Under Camera 2 (Autodesk Fusion 360 design; units mm, degrees)
Autodesk Fusion 360 part; units mm, degrees
note: some values were not read from the file. Chosen so that the rebuilt part matches the saved one: a direction. Set by a fixed rule: which sketch regions a step uses.
sketch "Sketch1" plane through (0, -227.1998, 566.5) normal (1, 0, 0) x (0, 1, 0) in component "Under Cam"
  line L0 (-26, -3.5) -> (12.5005, -3.5)
  line L1 (12.5005, -3.5) -> (4.8799, -38.213)
  line L2 (4.8799, -38.213) -> (-8.0595, -38.213)
  line L3 (-8.0595, -38.213) -> (-8.0595, -43.5)
  line L4 (-8.0595, -43.5) -> (-17.1111, -43.5)
  line L5 (-17.1111, -43.5) -> (-26, -3.5)
  dimension "d394" = 40
  dimension "d403" = 0
  dimension "d404" = 0
  dimension "d405" = 0
  dimension "d406" = 0
  dimension "d415" = 0
  dimension "d416" = 0
  dimension "d417" = 0
  dimension "d418" = 0
  dimension "d423" = 0
  dimension "d424" = 0
  dimension "d425" = 0
  dimension "d426" = 0
  dimension "d432" = 0
  dimension "d433" = 0
  dimension "d434" = 0
  dimension "d435" = 0
  dimension "d440" = 0
  dimension "d441" = 0
  dimension "d442" = 0
  dimension "d443" = 0
  constraint horizontal L0
  constraint parallel L0 L2
  constraint perpendicular L2 L3
  constraint perpendicular L3 L4
  measures "d394" distance of L0 L4
extrude "Extrude1" add sketch "Sketch1" against normal blind 32 makes body 1 in component "Under Cam"
ref_plane "WorkPlane2" through (-16, -253.2593, 525.6435) normal (0, 1, 0) x (0, 0, -1) in component "Under Cam"
sketch "Sketch2" plane through (-71.456, -253.2593, 540.4111) normal (0, 1, 0) x (1, 0, 0) in component "Under Cam"
  line L0 (71.456, 17.4112) -> (71.456, -22.5888)
  line L1 (71.456, -22.5888) -> (39.456, -22.5888)
  line L2 (39.456, -22.5888) -> (39.456, 17.4112)
  line L3 (39.456, 17.4112) -> (71.456, 17.4112)
  line L4 (41.456, -21.5888) -> (69.456, -21.5888)
  line L5 (69.456, -21.5888) -> (69.456, 17.4112)
  line L6 (69.456, 17.4112) -> (41.456, 17.4112)
  line L7 (41.456, 17.4112) -> (41.456, -21.5888)
  line L8 (41.456, -21.5888) -> (69.456, -21.5888)
  line L9 (69.456, -21.5888) -> (69.456, -22.5888)
  line L10 (69.456, -22.5888) -> (41.456, -22.5888)
  line L11 (41.456, -22.5888) -> (41.456, -21.5888)
  line L12 (41.456, -21.5888) -> (41.456, -22.5888)
  line L13 (69.456, -21.5888) -> (69.456, -22.5888)
  dimension "d273" = 2
  dimension "d274" = 2
  dimension "d275" = 1
  constraint horizontal L4
  constraint vertical L5
  constraint horizontal L6
  constraint vertical L7
  constraint coincident L3 L5.end
  constraint horizontal L8
  constraint vertical L9
  constraint horizontal L10
  constraint vertical L11
  constraint coincident L1 L9.end
  constraint perpendicular L10 L13
  measures "d273" horizontal distance of L1.end L4.start
  measures "d274" horizontal distance of L0.end L4.end
  measures "d275" vertical distance of L0.end L4.end
extrude "Extrude2" cut sketch "Sketch2" along normal blind 10 contours L3 L4 L5 L6 L7 L8 | L1 L4 L8 L9 L10 L11 L12 L13 bodies 1 in component "Under Cam"
sketch "Sketch8" plane through (0, 0, 563) normal (0, 0, 1) x (-1, 0, 0) in component "Under Cam"
  line L0 (0, 253.1998) -> (0, 214.6993)
  line L1 (0, 214.6993) -> (32, 214.6993)
  line L2 (32, 214.6993) -> (32, 253.1998)
  line L3 (2, 253.1998) -> (0, 253.1998)
  line L4 (20, 214.6965) -> (20, 253.2026) construction
  circle A0 centre (20, 226.9495) radius 0.75
  circle A1 centre (20, 240.9495) radius 0.75
  line L5 (20, 233.9495) -> (0, 233.9495) construction
  line L6 (30, 253.1998) -> (30, 243.2593)
  line L7 (30, 243.2593) -> (2, 243.2593)
  line L8 (2, 243.2593) -> (2, 253.1998)
  line L9 (32, 253.1998) -> (30, 253.1998)
  dimension "d389" = 1.5
  dimension "d390" = 1.5
  dimension "d391" = 7
  dimension "d392" = 7
  dimension "d427" = 12
  constraint coincident L4 A0.centre
  constraint coincident L4 A1.centre
  constraint midpoint L4 L5.start
  constraint midpoint L0 L5.end
  constraint perpendicular L3 L4
  constraint perpendicular L4 L5
  measures "d389" diameter of A0
  measures "d390" diameter of A1
  measures "d391" distance of A1.centre L5.start
  measures "d392" distance of A0.centre L5.start
  measures "d427" distance of L2 L4
extrude "Extrude11" cut sketch "Sketch8" against normal blind 10 contours A0 | A1 bodies 1 in component "Under Cam"
sketch "Sketch1 (2)" plane through (0, 0, 0) normal (0, 0, 1) x (1, 0, 0) in component "ESP32"
  line L0 (13.5, -20) -> (-13.5, -20)
  line L1 (-13.5, -20) -> (-13.5, 20)
  line L2 (-13.5, 20) -> (13.5, 20)
  line L3 (13.5, 20) -> (13.5, -20)
  line L4 (13.5, -20) -> (-13.5, 20) construction
  line L5 (-13.5, -20) -> (13.5, 20) construction
  dimension "d395" = 27
  dimension "d396" = 40
  dimension "d399" = 0
  dimension "d400" = 0
  dimension "d401" = 0
  dimension "d402" = 0
  dimension "d411" = 0
  dimension "d412" = 0
  dimension "d413" = 0
  dimension "d414" = 0
  dimension "d419" = 0
  dimension "d420" = 0
  dimension "d421" = 0
  dimension "d422" = 0
  dimension "d428" = 0
  dimension "d429" = 0
  dimension "d430" = 0
  dimension "d431" = 0
  dimension "d436" = 0
  dimension "d437" = 0
  dimension "d438" = 0
  dimension "d439" = 0
  constraint perpendicular L0 L1
  constraint parallel L0 L2
  constraint parallel L1 L3
  constraint horizontal L0
  constraint coincident L4 origin
  constraint coincident L5 origin
  measures "d395" distance of L1.end L2.end
  measures "d396" distance of L0.end L1.end
extrude "Extrude1'" add sketch "Sketch1 (2)" along normal blind 18 separate body makes body 2 in component "ESP32"
sketch "Sketch9" plane through (0, 0, 523) normal (0, 0, -1) x (1, 0, 0) in component "Under Cam"
  line L0 (-30, 243.2593) -> (-30, 244.3109)
  line L1 (-30, 244.3109) -> (-32, 244.3109)
  line L2 (-32, 244.3109) -> (-32, 235.2593)
  line L3 (-32, 235.2593) -> (0, 235.2593)
  line L4 (0, 235.2593) -> (0, 244.3109)
  line L5 (0, 244.3109) -> (-2, 244.3109)
  line L6 (-2, 244.3109) -> (-2, 243.2593)
  line L7 (-2, 243.2593) -> (-30, 243.2593)
  line L8 (0, 222.3199) -> (0, 235.2593)
  line L9 (0, 235.2593) -> (-32, 235.2593)
  line L10 (-32, 235.2593) -> (-32, 222.3199)
  line L11 (-32, 222.3199) -> (0, 222.3199)
  line L12 (-32, 241.2593) -> (0, 241.2593)
  line L13 (0, 241.2593) -> (0, 222.3199)
  line L14 (0, 222.3199) -> (-32, 222.3199)
  line L15 (-32, 222.3199) -> (-32, 241.2593)
  line L16 (-32, 222.3199) -> (0, 222.3199)
  line L17 (0, 222.3199) -> (0, 212.3199)
  line L18 (0, 212.3199) -> (-32, 212.3199)
  line L19 (-32, 212.3199) -> (-32, 222.3199)
  line L20 (-32, 241.2593) -> (-29, 241.2593)
  line L21 (-29, 241.2593) -> (-29, 212.3199)
  line L22 (-29, 212.3199) -> (-32, 212.3199)
  line L23 (-32, 212.3199) -> (-32, 241.2593)
  dimension "d452" = 2
  dimension "d455" = 10
  dimension "d456" = 3
  constraint horizontal L12
  constraint vertical L13
  constraint horizontal L14
  constraint vertical L15
  constraint coincident L8.start L11.end
  constraint coincident L2 L12.start
  constraint horizontal L16
  constraint vertical L17
  constraint horizontal L18
  constraint vertical L19
  constraint coincident L10.end L11.start
  constraint horizontal L20
  constraint vertical L21
  constraint horizontal L22
  constraint vertical L23
  constraint coincident L18 L21.end
  measures "d452" distance of L7 L12
  measures "d455" distance of L10.end L18.end
  measures "d456" distance of L12.start L20.end
extrude "Extrude12" cut sketch "Sketch9" against normal blind 28 contours L3 L4 L9 L12 L13 L21 | L3 L8 L9 L11 L13 L14 L16 L21 | L11 L14 L16 L17 L18 L21 bodies 1 in component "Under Cam"
fillet "Fillet1" radius 10 1 edges at (-14.5, -241.2593, 551) on bodies 1 in component "Under Cam"
sketch "Sketch10" plane through (0, -243.2593, 0) normal (0, -1, 0) x (1, 0, 0) in component "Under Cam"
  line L0 (-30, 523) -> (-2, 523)
  line L1 (-2, 523) -> (-2, 563)
  line L2 (-2, 563) -> (-30, 563)
  line L3 (-30, 563) -> (-30, 523)
  circle A0 centre (-16, 555) radius 2.5
  dimension "d458" = 5
  dimension "d459" = 8
  measures "d458" diameter of A0
  measures "d459" distance of L2 A0.centre
extrude "Extrude13" cut sketch "Sketch10" against normal through all contours A0 bodies 1 in component "Under Cam"
component "Under Cam" placed x (1, 0, 0) y (0, 1, 0) z (0, 0, 1) at (0, 0, 0)
component "ESP32" placed x (-1, 0, 0) y (0, 0, 1) z (0, 1, 0) at (-16, -261.2593, 543)
equation "Trous_Vis_diam2 = 2.2 mm"
named bodies: "support double cam"
